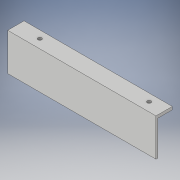
# Autodesk Inventor part: Camera Mount
Saved by Autodesk Inventor 2018.1 (Build 221171000, 171)
## iProperties
Created: 2017-11-17
Part Number: Camera Mount
Material: Generic
Document SubType Name: Modeling
Designer: trenton.fender
Density: 1 g/cm^3
Appearance: Default
Author: trenton.fender
Autodesk Inventor part; units mm, degrees
ref_plane "YZ Plane" through (0, 0, 0) normal (1, 0, 0) x (0, 1, 0)
ref_plane "XZ Plane" through (0, 0, 0) normal (0, 1, 0) x (-1, 0, 0)
ref_plane "XY Plane" through (0, 0, 0) normal (0, 0, 1) x (1, 0, 0)
sketch "Sketch1" plane through (0, 0, 0) normal (0, 0, 1) x (1, 0, 0)
  line L0 (0, 0) -> (241.3, 0)
  line L1 (241.3, 0) -> (241.3, 60.96)
  line L2 (241.3, 60.96) -> (0, 60.96)
  line L3 (0, 60.96) -> (0, 0)
  dimension "d0" = 241.3
  dimension "d1" = 60.96
  constraints: 8 end point, 2 parallel, 1 horizontal, 1 perpendicular
  measures "d0" distance of L1.end L2.end
  measures "d1" distance of L0.end L1.end
extrude "Extrusion1" add sketch "Sketch1" along normal blind 3.175
sketch "Sketch2" plane through (0, 0, 0) normal (0, 0, -1) x (-1, 0, 0)
  line L0 (-241.3, 60.96) -> (0, 60.96) projected
  line L1 (-241.3, 0) -> (-241.3, 60.96) projected
  line L2 (0, 60.96) -> (-241.3, 60.96)
  line L3 (-241.3, 60.96) -> (-241.3, 56.1975)
  line L4 (-241.3, 56.1975) -> (0, 56.1975)
  line L5 (0, 56.1975) -> (0, 60.96)
  point P0 (0, 0)
  dimension "d4" = 4.7625
  constraints: 8 end point, 2 parallel, 1 horizontal, 1 perpendicular, 1 point on line
  measures "d4" distance of L3.end L2.end
extrude "Extrusion2" add sketch "Sketch2" along normal blind 23.495
sketch "Sketch3" plane through (0, 60.96, 3.175) normal (0, 1, 0) x (1, 0, 0)
  circle A0 centre (38.1, 14.2875) radius 3.0988
  circle A1 centre (215.9, 14.2875) radius 3.0988
  line L0 (241.3, 26.67) -> (241.3, 0) projected
  line L1 (0, 26.67) -> (241.3, 26.67) projected
  point P0 (0, 3.175)
  dimension "d7" = 6.1976
  dimension "d8" = 6.1976
  dimension "d9" = 177.8
  dimension "d10" = 25.4
  dimension "d11" = 12.3825
  dimension "d12" = 12.3825
  constraints: 2 centre point
  measures "d7" diameter of A0
  measures "d8" diameter of A1
  measures "d9" distance of A1.centre A0.centre
  measures "d10" distance from line of L0 A1.centre
  measures "d11" distance from line of L1 A1.centre
  measures "d12" distance from line of L1 A0.centre
extrude "Extrusion3" cut sketch "Sketch3" against normal blind 6.1976
equation "\"d12\" = d11"
equation "\"d13\" = d8"
body "Solid1"
